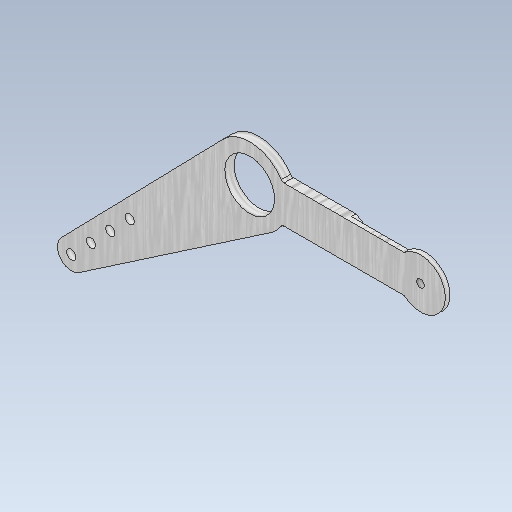
# Autodesk Inventor part: アーム中間節test
Saved by Autodesk Inventor 2020.2 (Build 242310000, 310)
## iProperties
Created: 2020-02-28
Part Number: アーム中間節test
Material: アルミニウム 7075
Document SubType Name: Modeling
Designer: aoyam
Density: 2.81 g/cm^3
Appearance: サテン - ブラシ仕上げ 重厚
Mass: 12.7352 g
Surface Area: 52.8345 cm^2
Volume: 4.53211 cm^3
Author: aoyam
Autodesk Inventor part; units mm, degrees
ref_plane "YZ Plane" through (0, 0, 0) normal (1, 0, 0) x (0, 1, 0)
ref_plane "XZ Plane" through (0, 0, 0) normal (0, 1, 0) x (-1, 0, 0)
ref_plane "XY Plane" through (0, 0, 0) normal (0, 0, 1) x (1, 0, 0)
sketch "スケッチ1" plane through (0, 0, 0) normal (0, 0, 1) x (1, 0, 0)
  circle A0 centre (-55, 0) radius 8.025
  line L0 (6, -6) -> (-61, -6)
  line L1 (-61, -6) -> (-61, 6)
  line L2 (-61, 6) -> (6, 6)
  line L3 (-61, -6) -> (-61, 6)
  line L4 (-20.8557, 4.9841) -> (202.5072, 4.9841) construction
  circle A1 centre (0, 0) radius 8
  line L5 (-23.9175, 26.3005) -> (3.7655, 4.6721)
  circle A2 centre (0, 0) radius 1.25
  circle A3 centre (0, 0) radius 3
  line L6 (-11, -6) -> (-9.3095, -2.3748)
  line L7 (-9.3095, -2.3748) -> (-23.8151, 6)
  line L8 (0, 0) -> (0, -6)
  circle A4 centre (-55, 0) radius 8.025
  circle A5 centre (0, 0) radius 1.5
  arc A6 (-44.5788, 6) -> (-48.2949, 9.9821) centre (-55, 0) ccw
  line L9 (-44.5788, -6) -> (-5.2915, -6)
  arc A7 (-5.2915, -6) -> (-5.2915, 6) centre (0, 0) ccw
  line L10 (-5.2915, 6) -> (-44.5788, 6)
  line L11 (-55, 0) -> (0, 0)
  circle A8 centre (-55, 0) radius 8.025
  circle A9 centre (0, 0) radius 1.5
  arc A10 (-44.5788, 6) -> (-48.1673, 9.8952) centre (-55, 0) ccw
  line L12 (-44.5788, -6) -> (-5.2915, -6)
  arc A11 (-5.2915, -6) -> (-5.2915, 6) centre (0, 0) ccw
  line L13 (-5.2915, 6) -> (-44.5788, 6)
  circle A12 centre (-55, 0) radius 8.025
  line L14 (-61, 6) -> (-61, -6)
  line L15 (-61, 6) -> (-61, -6)
  circle A13 centre (-55, 0) radius 8.025
  arc A14 (-48.2949, -9.9821) -> (-44.5788, -6) centre (-55, 0) ccw
  arc A15 (-44.5788, 6) -> (-63.6661, 8.3366) centre (-55, 0) ccw
  circle A16 centre (-55, 0) radius 8.025
  arc A17 (-48.1673, -9.8952) -> (-44.5788, -6) centre (-55, 0) ccw
  arc A18 (-44.5788, 6) -> (-63.5584, 8.4472) centre (-55, 0) ccw
  circle A19 centre (-55, 0) radius 8.025
  circle A20 centre (0, 0) radius 1.5
  arc A21 (-44.5788, 6) -> (-48.2337, 9.9407) centre (-55, 0) ccw
  line L16 (-48.2337, 9.9407) -> (-109.9213, 51.9291)
  arc A22 (-109.9213, 51.9291) -> (-115.6772, 45.0695) centre (-112.4533, 48.2091) ccw
  line L17 (-115.6772, 45.0695) -> (-63.6148, -8.3897)
  arc A23 (-63.6148, -8.3897) -> (-44.5788, -6) centre (-55, 0) ccw
  line L18 (-44.5788, -6) -> (-5.2915, -6)
  arc A24 (-5.2915, -6) -> (-5.2915, 6) centre (0, 0) ccw
  line L19 (-5.2915, 6) -> (-44.5788, 6)
  circle A25 centre (-112.4533, 48.2091) radius 1.5
  circle A26 centre (-93.6158, 28.8662) radius 1.5
  circle A27 centre (-99.895, 35.3138) radius 1.5
  circle A28 centre (-106.1742, 41.7614) radius 1.5
  line L20 (-48.2337, -9.9407) -> (-109.9213, -51.9291)
  arc A29 (-115.6772, -45.0695) -> (-109.9213, -51.9291) centre (-112.4533, -48.2091) ccw
  line L21 (-115.6772, -45.0695) -> (-63.6148, 8.3897)
  circle A30 centre (-112.4533, -48.2091) radius 1.5
  circle A31 centre (-93.6158, -28.8662) radius 1.5
  circle A32 centre (-99.895, -35.3138) radius 1.5
  circle A33 centre (-106.1742, -41.7614) radius 1.5
  circle A34 centre (-55, 0) radius 11
  circle A35 centre (-57.5491, -13.2572) radius 1.5
  circle A36 centre (-57.5491, -13.2572) radius 2.5
  point P0 (-5.2915, 6)
  point P1 (-5.2915, -6)
  point P2 (-49.6708, 6)
  point P3 (-49.6708, -6)
  point P4 (-60.3292, -6)
  point P5 (-61, -5.3292)
  point P6 (-61, 5.3292)
  point P7 (-60.3292, 6)
  point P8 (5.2915, -6)
  point P9 (5.2915, 6)
  point P10 (-63.6661, -8.3366)
  point P11 (-44.5788, 6)
  point P12 (-48.2949, 9.9821)
  point P13 (-63.6148, 8.3897)
  point P14 (-57.5228, -11.7574)
  point P15 (-57.0173, -11.8546)
  dimension "d1" = 16.05
  dimension "d19" = 38
  dimension "d35" = 16
  dimension "d36" = 2.5
  dimension "d37" = 6
  dimension "d40" = 6
  dimension "d41" = 12
  dimension "d42" = 11
  dimension "d43" = 4
  dimension "d45" = 30
  dimension "d46" = 65
  dimension "d59" = 22
  dimension "d60" = 3
  dimension "d61" = 1
  constraints: 44 end point, 37 centre point, 26 point on circle, 19 symmetric about line, 4 coincident, 3 concentric, 3 point on line, 2 horizontal, 2 perpendicular, 2 tangent, 1 parallel, 25 other
  measures "d1" diameter of A0
  measures "d19" angle of L2 L5
  measures "d35" diameter of A1
  measures "d36" diameter of A2
  measures "d37" diameter of A3
  measures "d40" distance of L8.start L8.end
  measures "d41" distance between parallel lines of L2 L0
  measures "d42" distance of L8.end L6.start
  measures "d43" distance of L6.start L6.end
  measures "d45" angle of L2 L7
  measures "d46" angle of L0 L6
  measures "d59" diameter of A34
  measures "d60" diameter of A35
  measures "d61" radial gap between concentric circles of A35 A36
extrude "押し出し1" add sketch "スケッチ1" along normal blind 3 contours L11 A34 L0 A0 | A0 L2 A34 L11 | A0 L2 L1 L0 A34 | A34 L2 L7 L11 | L11 L7 L6 L0 A34 | A0 L1 L2 | A34 A36 A23 L17 L21 A15 A6 L2 | L0 L1 A0 | L0 A14 A23 A36 A34 | L11 A1 L0 L6 L7 | L7 L2 A1 L11 | A36 A23 A35 | L11 A3 L8 L0 A1 | A1 L2 L0 L8 A3 L11 | A36 A23 A35 | A23 L20 A36 | A36 L20 A29 L21 L17 A23 | A1 L5 L2 | L0 A1 | L11 A5 L8 A3 | A3 L8 A5 L11 | A35 A23 | A23 A35 | L5 A1 L2 | L11 A2 L8 A5 | A5 L8 A2 L11
extrude "押し出し3" cut sketch "スケッチ1" along normal blind 1.5 contours L11 A1 L0 L6 L7 | L7 L2 A1 L11 | L11 A3 L8 L0 A1 | A1 L2 L0 L8 A3 L11 | A1 L5 L2 | L0 A1 | L5 A1 L2
thread "ねじ4" size "M3x0.5" class "6H" standard "ANSI Metric M Profile" full length
sketch "スケッチ2" plane through (0, 0, 3) normal (0, 0, 1) x (1, 0, 0)
  circle A0 centre (0, 0) radius 1.25 projected
  arc A1 (-5.2915, -6) -> (-5.2915, 6) centre (0, 0) ccw projected
  line L0 (-5.2915, 6) -> (-44.5788, 6) projected
  circle A2 centre (-55, 0) radius 8.025 projected
  line L1 (-44.5788, -6) -> (-5.2915, -6) projected
  arc A3 (-44.5788, 6) -> (-63.6148, 8.3897) centre (-55, 0) ccw projected
  line L2 (-63.6148, 8.3897) -> (-115.6772, -45.0695) projected
  arc A4 (-115.6772, -45.0695) -> (-109.9213, -51.9291) centre (-112.4533, -48.2091) ccw projected
  line L3 (-109.9213, -51.9291) -> (-48.2337, -9.9407) projected
  arc A5 (-48.2337, -9.9407) -> (-44.5788, -6) centre (-55, 0) ccw projected
sketch "スケッチ4" plane through (0, 0, 0) normal (0, 0, -1) x (-1, 0, 0)
  line L0 (9.3095, -2.3748) -> (11, -6) projected
  line L1 (23.8151, 6) -> (9.3095, -2.3748) projected
  circle A0 centre (55, 0) radius 12.025
  arc A1 (47.626, -1.5) -> (50.8041, -6.2466) centre (55, 0) ccw
  line L2 (47.626, -1.5) -> (19.8247, -1.5)
  line L3 (19.8247, -1.5) -> (25.0208, 1.5)
  line L4 (25.0208, 1.5) -> (47.626, 1.5)
  arc A2 (60.4231, 5.2169) -> (47.626, 1.5) centre (55, 0) ccw
  line L5 (60.4231, 5.2169) -> (105.9193, -42.0773)
  arc A3 (105.2801, -42.839) -> (105.9193, -42.0773) centre (105.5589, -42.424) ccw
  line L6 (105.2801, -42.839) -> (50.8041, -6.2466)
  circle A4 centre (84.7607, -20.8038) radius 4.5
  circle A5 centre (79.3836, -23.5767) radius 1.55
  line L7 (22.4227, 0) -> (40.2559, 0) construction
  line L8 (22.4227, -2) -> (40.2559, -2)
  line L9 (40.2559, 2) -> (22.4227, 2)
  arc A6 (22.4227, 2) -> (22.4227, -2) centre (22.4227, 0) ccw
  arc A7 (40.2559, -2) -> (40.2559, 2) centre (40.2559, 0) ccw
  line L10 (23.8151, 6) -> (44.5788, 6) projected
  circle A8 centre (55, 0) radius 8.025 projected
  line L11 (44.5788, -6) -> (11, -6) projected
  arc A9 (44.5788, -6) -> (48.2337, -9.9407) centre (55, 0) ccw projected
  line L12 (109.9213, -51.9291) -> (48.2337, -9.9407) projected
  arc A10 (109.9213, -51.9291) -> (115.6772, -45.0695) centre (112.4533, -48.2091) ccw projected
  line L13 (63.6148, 8.3897) -> (115.6772, -45.0695) projected
  arc A11 (63.6148, 8.3897) -> (44.5788, 6) centre (55, 0) ccw projected
  point P0 (0, 0)
  point P1 (31.3393, 0)
  point P2 (80.7612, -22.8663)
  point P3 (82.0206, -17.2342)
  point P4 (66.9256, -1.5427)
  point P5 (58.5901, -11.4766)
  point P6 (78.5193, -24.8633)
  dimension "d54" = 3.1
  dimension "d55" = 4
  constraints: 18 end point, 10 point on circle, 8 centre point, 6 tangent, 2 midpoint, 1 parallel
  measures "d54" diameter of A5
  measures "d55" diameter of A7
extrude "押し出し4" cut sketch "スケッチ4" against normal blind 2.5 contours A0 L5 A4 A5 L6 | A7 L8 A6 L2 | L2 A6 L3 L4 A7 | L4 L3 A6 L9 A7 | A5
fillet "フィレット1" radius 1.05 5 edges at (-66.9256, -1.5427, 1.25) (-58.5901, -11.4766, 1.25) (-82.0206, -17.2342, 1.25) (-44.5788, -6, 1.5) (-44.5788, 6, 1.5)
sketch "スケッチ5" plane through (0, 0, 0) normal (0, 0, -1) x (-1, 0, 0)
  arc A0 (40.2559, -2) -> (40.2559, 2) centre (40.2559, 0) ccw projected
  line L0 (40.2559, -2) -> (22.4227, -2) projected
  arc A1 (22.4227, 2) -> (22.4227, -2) centre (22.4227, 0) ccw projected
  line L1 (22.4227, 2) -> (40.2559, 2) projected
  line L2 (9.3095, -2.3748) -> (11, -6) projected
  line L3 (23.8151, 6) -> (9.3095, -2.3748) projected
  line L4 (23.8151, 6) -> (43.9885, 6) projected
  circle A2 centre (55, 0) radius 8.025 projected
  line L5 (43.9885, -6) -> (11, -6) projected
  arc A3 (44.8728, -6.4838) -> (48.2337, -9.9407) centre (55, 0) ccw projected
  line L6 (109.9213, -51.9291) -> (48.2337, -9.9407) projected
  arc A4 (109.9213, -51.9291) -> (115.6772, -45.0695) centre (112.4533, -48.2091) ccw projected
  line L7 (63.6148, 8.3897) -> (115.6772, -45.0695) projected
  arc A5 (63.6148, 8.3897) -> (44.8728, 6.4838) centre (55, 0) ccw projected
  arc A6 (44.8728, -6.4838) -> (43.9885, -6) centre (43.9885, -7.05) ccw projected
  arc A7 (43.9885, 6) -> (44.8728, 6.4838) centre (43.9885, 7.05) ccw projected
  point P0 (0, 0)
